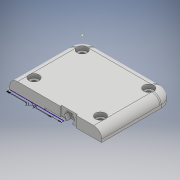
# Autodesk Inventor part: golova 3 krushka
Saved by Autodesk Inventor 2018.2 (Build 222227000, 227)
## iProperties
Created: 2026-01-20
Part Number: golova 3 krushka
Material: Типовые
Document SubType Name: Modeling
Designer: Denis
Density: 1 g/cm^3
Appearance: По умолчанию
Author: Denis
Autodesk Inventor part; units mm, degrees
ref_plane "YZ Plane" through (0, 0, 0) normal (1, 0, 0) x (0, 1, 0)
ref_plane "XZ Plane" through (0, 0, 0) normal (0, 1, 0) x (-1, 0, 0)
ref_plane "XY Plane" through (0, 0, 0) normal (0, 0, 1) x (1, 0, 0)
sketch "Эскиз1" plane through (0, 0, 0) normal (0, 0, 1) x (1, 0, 0)
  line L0 (0, 0) -> (64.3, 0)
  line L1 (64.3, 0) -> (64.3, -50.7)
  line L2 (64.3, -50.7) -> (0, -50.7)
  line L3 (0, -50.7) -> (0, 0)
  dimension "d0" = 64.3
  dimension "d1" = 50.7
  constraints: 8 end point, 2 parallel, 1 horizontal, 1 perpendicular
  measures "d0" distance of L1.end L2.end
  measures "d1" distance of L0.end L1.end
extrude "Выдавливание1" add sketch "Эскиз1" along normal blind 7.6
sketch "Эскиз2" plane through (0, -50.7, 0) normal (0, -1, 0) x (1, 0, 0)
  line L0 (0, 0) -> (64.3, 0) projected
  line L1 (0, 0) -> (32.15, 0)
  line L2 (32.15, 0) -> (33.95, 0)
  line L3 (33.95, 0) -> (35.75, 3.1177)
  line L4 (35.75, 3.1177) -> (33.95, 6.2354)
  line L5 (33.95, 6.2354) -> (30.35, 6.2354)
  line L6 (30.35, 6.2354) -> (28.55, 3.1177)
  line L7 (28.55, 3.1177) -> (30.35, 0)
  line L8 (30.35, 0) -> (32.15, 0)
  dimension "d4" = 32.15
  dimension "d5" = 1.8
  dimension "d6" = 3.6
  dimension "d7" = 120
  dimension "d8" = 3.6
  dimension "d9" = 120
  constraints: 16 end point, 2 point on line, 1 collinear, 1 horizontal, 1 midpoint
  measures "d4" distance of L0.start L1.end
  measures "d5" distance of L1.end L2.end
  measures "d6" distance of L2.end L3.end
  measures "d7" angle of L3 L2
  measures "d8" distance of L3.end L4.end
  measures "d9" angle of L4 L3
extrude "Выдавливание2" cut sketch "Эскиз2" against normal blind 3.8
sketch "Эскиз3" plane through (0, -50.7, 7.6) normal (0, -1, 0) x (1, 0, 0)
  circle A0 centre (32.15, -4.4823) radius 1.8
  point P0 (0, -7.6)
  dimension "d12" = 3.6
  constraints: 1 centre point
  measures "d12" diameter of A0
extrude "Выдавливание3" cut sketch "Эскиз3" against normal blind 6.8
sketch "Эскиз4" plane through (0, -50.7, 7.6) normal (0, -1, 0) x (1, 0, 0)
  circle A0 centre (32.15, -4.4823) radius 1.8 projected
  line L0 (32.15, -4.4823) -> (37.65, -4.4823)
  line L1 (64.3, -7.6) -> (33.95, -7.6) projected
  line L2 (0, 0) -> (64.3, 0) projected
  line L3 (37.65, -7.6) -> (26.65, -7.6)
  line L4 (26.65, -7.6) -> (26.65, 0)
  line L5 (26.65, 0) -> (37.65, 0)
  line L6 (37.65, 0) -> (37.65, -7.6)
  point P0 (0, -7.6)
  dimension "d15" = 5.5
  dimension "d16" = 11
  constraints: 10 end point, 2 horizontal, 2 parallel, 2 point on line, 1 perpendicular
  measures "d15" distance of L0.start L0.end
  measures "d16" distance of L4.end L5.end
extrude "Выдавливание4" cut sketch "Эскиз4" against normal blind 1
fillet "Сопряжение1" radius 9 2 edges at (0, 0, 3.8) (64.3, 0, 3.8)
sketch "Эскиз5" plane through (0, 0, 7.6) normal (0, 0, 1) x (1, 0, 0)
  line L0 (0, 0) -> (8.864, -0.001)
  arc A0 (9, 0) -> (0, -9) centre (9, -9) ccw projected
  line L1 (8.864, -0.001) -> (8.863, -8.865)
  circle A1 centre (8.863, -8.865) radius 1.8
  line L2 (64.3, 0) -> (55.436, 0)
  line L3 (55.3, 0) -> (9, 0) projected
  line L4 (55.436, 0) -> (55.436, -8.864)
  circle A2 centre (55.436, -8.864) radius 1.8
  dimension "d20" = 8.864
  dimension "d21" = 8.864
  dimension "d22" = 3.6
  dimension "d23" = 8.864
  dimension "d24" = 8.864
  dimension "d25" = 90
  dimension "d26" = 3.6
  constraints: 8 end point, 2 centre point, 2 coincident, 2 perpendicular, 1 collinear, 1 point on circle
  measures "d20" distance of L0.start L0.end
  measures "d21" distance of L0.end L1.end
  measures "d22" diameter of A1
  measures "d23" distance of L2.start L2.end
  measures "d24" distance of L2.end L4.end
  measures "d25" angle of L4 L2
  measures "d26" diameter of A2
extrude "Выдавливание5" cut sketch "Эскиз5" against normal blind 10
sketch "Эскиз6" plane through (0, 0, 7.6) normal (0, 0, 1) x (1, 0, 0)
  circle A0 centre (8.863, -8.865) radius 1.8 projected
  line L0 (8.863, -8.865) -> (8.863, -42.636)
  circle A1 centre (8.863, -42.636) radius 1.8
  circle A2 centre (55.436, -8.864) radius 1.8 projected
  line L1 (55.436, -8.864) -> (55.436, -42.635)
  circle A3 centre (55.436, -42.635) radius 1.8
  point P0 (0, 0)
  dimension "d29" = 33.771
  dimension "d30" = 3.6
  dimension "d31" = 33.771
  dimension "d32" = 3.6
  constraints: 4 end point, 2 centre point, 2 coincident, 2 vertical
  measures "d29" distance of L0.start L0.end
  measures "d30" diameter of A1
  measures "d31" distance of L1.start L1.end
  measures "d32" diameter of A3
extrude "Выдавливание6" cut sketch "Эскиз6" against normal blind 10 contours A1 | A3
sketch "Эскиз7" plane through (0, 0, 7.6) normal (0, 0, 1) x (1, 0, 0)
  point P0 (0, 0)
sketch "Эскиз8" plane through (0, 0, 7.6) normal (0, 0, 1) x (1, 0, 0)
  circle A0 centre (8.863, -8.865) radius 1.8 projected
  circle A1 centre (8.863, -8.865) radius 3.55
  circle A2 centre (55.436, -8.864) radius 1.8 projected
  circle A3 centre (55.436, -8.864) radius 3.55
  circle A4 centre (55.436, -42.635) radius 1.8 projected
  circle A5 centre (55.436, -42.635) radius 3.55
  circle A6 centre (8.863, -42.636) radius 1.8 projected
  circle A7 centre (8.863, -42.636) radius 3.55
  point P0 (0, 0)
  dimension "d35" = 7.1
  dimension "d36" = 7.1
  dimension "d37" = 7.1
  dimension "d38" = 7.1
  constraints: 4 centre point, 4 coincident
  measures "d35" diameter of A1
  measures "d36" diameter of A3
  measures "d37" diameter of A5
  measures "d38" diameter of A7
extrude "Выдавливание7" cut sketch "Эскиз8" against normal blind 2.8
fillet "Сопряжение2" radius 5.5 5 edges at (2.636, -2.636, 7.6) (32.15, 0, 7.6) (61.664, -2.636, 7.6) (64.3, -29.85, 7.6) (0, -29.85, 7.6)
sketch "Эскиз9" plane through (0, 0, 0) normal (0, 0, -1) x (-1, 0, 0)
  line L0 (0, -50.7) -> (0, -9) projected
  line L1 (0, -50.7) -> (-31.3, -50.7)
  line L2 (-26.65, -50.7) -> (0, -50.7) projected
  point P0 (0, 0)
  dimension "d42" = 31.3
  constraints: 2 end point, 1 collinear
  measures "d42" distance of L0.start L1.end
sketch "Эскиз10" plane through (37.65, -50.7, 0) normal (0, -1, 0) x (1, 0, 0)
  point P0 (-37.65, 0)
sketch "Эскиз11" plane through (0, -49.7, 7.6) normal (0, -1, 0) x (1, 0, 0)
  line L0 (9, -7.6) -> (55.3, -7.6) projected
  line L1 (36.8968, -7.6) -> (28.1351, -7.6)
  line L2 (28.1351, -7.6) -> (28.1351, -0.8108)
  line L3 (28.1351, -0.8108) -> (36.8968, -0.8108)
  line L4 (36.8968, -0.8108) -> (36.8968, -7.6)
  point P0 (0, -7.6)
  constraints: 8 end point, 2 parallel, 1 horizontal, 1 perpendicular, 1 point on line
extrude "Выдавливание8" add sketch "Эскиз11" against normal blind 6.8
sketch "Эскиз12" plane through (37.65, -50.7, 0) normal (0, -1, 0) x (1, 0, 0)
  line L0 (0, 7.6) -> (0, 0) projected
  line L1 (26.65, 0) -> (0, 0) projected
  line L2 (0, 7.6) -> (6, 7.6)
  line L3 (6, 7.6) -> (6, 0)
  line L4 (6, 0) -> (0, 0)
  line L5 (0, 0) -> (0, 7.6)
  point P0 (-37.65, 0)
  dimension "d45" = 6
  constraints: 8 end point, 2 parallel, 1 horizontal, 1 perpendicular, 1 point on line
  measures "d45" distance of L3.end L4.end
extrude "Выдавливание9" cut sketch "Эскиз12" against normal blind 1
sketch "Эскиз13" plane through (0, -49.7, 7.6) normal (0, -1, 0) x (1, 0, 0)
  line L0 (26.65, -7.6) -> (0, -7.6) projected
  line L1 (0, -7.6) -> (31.3, -7.6)
  line L2 (31.3, -7.6) -> (33.1, -7.6)
  line L3 (9, -7.6) -> (55.3, -7.6) projected
  line L4 (43.65, 0) -> (43.65, -7.6) projected
  line L5 (64.3, -7.6) -> (43.65, -7.6) projected
  line L6 (43.65, 0) -> (47.65, 0)
  line L7 (47.65, 0) -> (47.65, -7.6)
  line L8 (47.65, -7.6) -> (43.65, -7.6)
  line L9 (43.65, -7.6) -> (43.65, 0)
  dimension "d48" = 31.3
  dimension "d49" = 1.8
  dimension "d50" = 4
  constraints: 12 end point, 2 parallel, 2 point on line, 1 collinear, 1 horizontal, 1 perpendicular
  measures "d48" distance of L0.end L1.end
  measures "d49" distance of L1.end L2.end
  measures "d50" distance of L7.end L8.end
extrude "Выдавливание10" cut sketch "Эскиз13" along normal blind 1
sketch "Эскиз14" plane through (0, -49.7, 7.6) normal (0, -1, 0) x (1, 0, 0)
  line L0 (0, -7.6) -> (37.3, -7.6)
  line L1 (9, -7.6) -> (55.3, -7.6) projected
  line L2 (37.3, -7.6) -> (39.1, -7.6)
  line L3 (39.1, -7.6) -> (42.7, -7.6)
  line L4 (42.7, -7.6) -> (44.5, -4.4823)
  line L5 (44.5, -4.4823) -> (42.7, -1.3646)
  line L6 (42.7, -1.3646) -> (39.1, -1.3646)
  line L7 (39.1, -1.3646) -> (37.3, -4.4823)
  line L8 (37.3, -4.4823) -> (39.1, -7.6)
  dimension "d53" = 37.3
  dimension "d54" = 1.8
  dimension "d55" = 3.6
  dimension "d56" = 3.6
  dimension "d57" = 120
  dimension "d58" = 3.6
  dimension "d59" = 120
  constraints: 16 end point, 3 parallel, 3 point on line
  measures "d53" distance of L0.start L0.end
  measures "d54" distance of L0.end L2.end
  measures "d55" distance of L2.end L3.end
  measures "d56" distance of L3.end L4.end
  measures "d57" angle of L4 L3
  measures "d58" distance of L4.end L5.end
  measures "d59" angle of L5 L4
extrude "Выдавливание11" cut sketch "Эскиз14" against normal blind 2.8
sketch "Эскиз15" plane through (0, -49.7, 7.6) normal (0, -1, 0) x (1, 0, 0)
  circle A0 centre (40.9, -4.4823) radius 1.8
  point P0 (0, -7.6)
  dimension "d62" = 3.6
  constraints: 1 centre point
  measures "d62" diameter of A0
extrude "Выдавливание12" cut sketch "Эскиз15" against normal blind 6.8
sketch "Эскиз16" plane through (0, -49.7, 7.6) normal (0, -1, 0) x (1, 0, 0)
  circle A0 centre (40.9, -4.4823) radius 1.8 projected
  line L0 (40.9, -4.4823) -> (46.4, -4.4823)
  line L1 (47.65, -7.6) -> (47.65, 0) projected
  line L2 (46.4, -7.6) -> (47.65, -7.6)
  line L3 (47.65, -7.6) -> (47.65, 0)
  line L4 (47.65, 0) -> (46.4, 0)
  line L5 (46.4, 0) -> (46.4, -7.6)
  point P0 (0, -7.6)
  dimension "d65" = 5.5
  constraints: 10 end point, 2 parallel, 2 perpendicular, 1 horizontal
  measures "d65" distance of L0.start L0.end
extrude "Выдавливание13" add sketch "Эскиз16" along normal blind 1 contours L5 L4 L1 L2
sketch "Эскиз17" plane through (0, -49.7, 7.6) normal (0, -1, 0) x (1, 0, 0)
  circle A0 centre (40.9, -4.4823) radius 1.8 projected
  line L0 (40.9, -4.4823) -> (46.4, -4.4823)
  line L1 (46.4, 0) -> (46.4, -7.6) projected
  line L2 (40.9, -4.4823) -> (35.4, -4.4823)
  line L3 (26.65, -7.6) -> (26.65, 0) projected
  line L4 (26.65, 0) -> (35.4, 0)
  line L5 (35.4, 0) -> (35.4, -7.6)
  line L6 (35.4, -7.6) -> (26.65, -7.6)
  line L7 (26.65, -7.6) -> (26.65, 0)
  point P0 (0, -7.6)
  dimension "d68" = 5.5
  dimension "d69" = 5.5
  constraints: 12 end point, 2 horizontal, 2 parallel, 1 perpendicular, 1 point on line
  measures "d68" distance of L0.start L0.end
  measures "d69" distance of L0.start L2.end
extrude "Выдавливание14" add sketch "Эскиз17" along normal blind 1 contours L5 L6 L3 L4
sketch "Эскиз18" plane through (0, 0, 0) normal (0, 0, -1) x (-1, 0, 0)
  line L0 (0, -50.7) -> (-38, -50.7)
  point P0 (0, 0)
  dimension "d72" = 38
  constraints: 2 end point, 1 horizontal
  measures "d72" distance of L0.start L0.end
sketch "Эскиз19" plane through (0, 0, 0) normal (0, 0, -1) x (-1, 0, 0)
  line L0 (0, -50.7) -> (-38, -50.7)
  line L1 (-38, -50.7) -> (-24.6, -50.7)
  line L2 (-24.6, -50.7) -> (-24.6, -48.7)
  line L3 (-24.6, -48.7) -> (-38, -48.7)
  line L4 (-38, -48.7) -> (-38, -50.7)
  point P0 (0, 0)
  dimension "d73" = 38
  dimension "d74" = 13.4
  dimension "d75" = 2
  constraints: 10 end point, 2 horizontal, 2 parallel, 1 perpendicular
  measures "d73" distance of L0.start L0.end
  measures "d74" distance of L3.end L2.end
  measures "d75" distance of L2.end L1.end
extrude "Выдавливание15" cut sketch "Эскиз19" against normal blind 1.2
